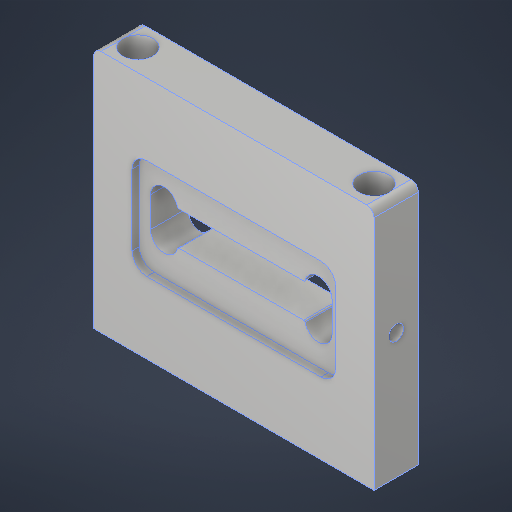
# Autodesk Inventor part: Spulenhalter Hinten Einzel
Saved by Autodesk Inventor 2025.2 (Build 292293000, 293)
## iProperties
Part Number: Spulenhalter Hinten Einzel
Material: Aluminium 6061
Document SubType Name: Modeling
Designer: rYan
Density: 2.7 g/cm^3
Appearance: Aluminium - flach
Mass: 16.9891 g
Surface Area: 44.1608 cm^2
Volume: 6.29226 cm^3
Author: rYan
Autodesk Inventor part; units mm, degrees
ref_plane "YZ Plane" through (0, 0, 0) normal (1, 0, 0) x (0, 1, 0)
ref_plane "XZ Plane" through (0, 0, 0) normal (0, 1, 0) x (-1, 0, 0)
ref_plane "XY Plane" through (0, 0, 0) normal (0, 0, 1) x (1, 0, 0)
sketch "Skizze1" plane through (0, 0, 0) normal (0, 1, 0) x (-1, 0, 0)
  line L0 (-19, 0) -> (-19, 30)
  line L1 (19, 30) -> (19, 0)
  line L2 (8.85, 11.45) -> (-8.85, 11.45)
  line L3 (-12.05, 11.45) -> (-12.05, 15.55)
  line L4 (-8.85, 15.55) -> (8.85, 15.55)
  line L5 (12.05, 15.55) -> (12.05, 11.45)
  arc A0 (12.05, 15.55) -> (8.85, 15.55) centre (10.45, 15.55) ccw
  arc A1 (8.85, 11.45) -> (12.05, 11.45) centre (10.45, 11.45) ccw
  arc A2 (-8.85, 15.55) -> (-12.05, 15.55) centre (-10.45, 15.55) ccw
  arc A3 (-12.05, 11.45) -> (-8.85, 11.45) centre (-10.45, 11.45) ccw
  line L6 (19, -3) -> (-19, -3)
  line L7 (-19, -3) -> (-19, 0)
  line L8 (19, 0) -> (19, -3)
  line L9 (0, 30) -> (19, 30)
  line L10 (19, 30) -> (-19, 30)
  arc A4 (-12.3, 11.45) -> (-8.617, 11.2) centre (-10.45, 11.45) ccw
  line L11 (-8.617, 11.2) -> (8.617, 11.2)
  arc A5 (8.617, 11.2) -> (12.3, 11.45) centre (10.45, 11.45) ccw
  line L12 (12.3, 11.45) -> (12.3, 15.55)
  arc A6 (12.3, 15.55) -> (8.617, 15.8) centre (10.45, 15.55) ccw
  line L13 (8.617, 15.8) -> (-8.617, 15.8)
  arc A7 (-8.617, 15.8) -> (-12.3, 15.55) centre (-10.45, 15.55) ccw
  line L14 (-12.3, 15.55) -> (-12.3, 11.45)
  line L15 (0, -3) -> (0, 30) construction
  point P0 (0, 13.5)
  point P1 (19, 0)
  point P2 (0, 13.5)
  dimension "d94" = 0.25
  constraints: 32 end point, 16 point on circle, 8 centre point, 6 parallel, 4 perpendicular, 4 tangent, 3 point on line, 2 horizontal, 2 midpoint, 6 other
  measures "d94" distance between parallel lines of L4 L13
extrude "Grundkörper" add sketch "Skizze1" along normal mid plane 6 contours L0 L10 L9 L1 L8 L6 L7
sketch "Skizze10" plane through (19, 3, -3) normal (0, 0, -1) x (-1, 0, 0)
  line L0 (-3.4, -3) -> (41.4, -3)
  line L1 (19, 19.4) -> (19, -25.4)
  point P0 (19, -3)
  point P1 (19, -3)
  point P2 (3, -3)
  point P3 (35, -3)
  dimension "d96" = 32
  constraints: 4 end point, 2 point on line, 1 symmetric about line
  measures "d96" distance of point (35, -3) point (3, -3)
hole "Fixierung" at (16, 0, -3) at (-16, 0, -3) direction (0, 0, 1) diameter 4.2 depth 8 tip angle 118
fillet "Rundung1" radius 1 2 edges at (-19, 0, 30) (19, 0, 30)
fillet "Rundung2" radius 0.2 4 edges at (-8.617, 0, 15.8) (8.617, 0, 15.8) (8.617, 0, 11.2) (-8.617, 0, 11.2)
sketch "Skizze13" plane through (0, -3, 0) normal (0, -1, 0) x (1, 0, 0)
  line L0 (-8.6611, 15.55) -> (8.6611, 15.55) construction
  line L1 (0, 15.55) -> (0, 11.45) construction
  line L2 (-8.6611, 11.45) -> (8.6611, 11.45) construction
  line L3 (-11.8, 6.7) -> (11.8, 6.7)
  line L4 (13.8, 8.7) -> (13.8, 18.3)
  line L5 (11.8, 20.3) -> (-11.8, 20.3)
  line L6 (-13.8, 18.3) -> (-13.8, 8.7)
  line L7 (-13.8, 6.7) -> (13.8, 20.3) construction
  line L8 (13.8, 6.7) -> (-13.8, 20.3) construction
  arc A0 (-11.8, 20.3) -> (-13.8, 18.3) centre (-11.8, 18.3) ccw
  arc A1 (-13.8, 8.7) -> (-11.8, 6.7) centre (-11.8, 8.7) ccw
  arc A2 (11.8, 6.7) -> (13.8, 8.7) centre (11.8, 8.7) ccw
  arc A3 (13.8, 18.3) -> (11.8, 20.3) centre (11.8, 18.3) ccw
  point P0 (0, 0)
  point P1 (0, 13.5)
  dimension "d125" = 27.6
  dimension "d126" = 13.6
  dimension "d127" = 2
  constraints: 14 end point, 8 point on circle, 8 point on line, 8 tangent, 5 midpoint, 4 centre point, 3 equal radius, 2 parallel, 1 horizontal, 1 perpendicular
  measures "d125" distance of L8.end L7.end
  measures "d126" distance of L7.end L8.start
  measures "d127" radius of A0
extrude "Tasche" cut sketch "Skizze13" against normal blind 1
sketch "Skizze11" plane through (19, -3, -3) normal (1, 0, 0) x (0, 0, -1)
  point P0 (-7, 3)
  point P1 (-17, 3)
hole "Federn" at (19, 0, 14) direction (-1, 0, 0) diameter 2 depth 4 tip angle 118
mirror "Spiegeln1" about plane through (0, 0, 0) normal (1, 0, 0) of "Federn"
sketch "Skizze12" plane through (-18, 3, 30) normal (0, 0, 1) x (1, 0, 0)
  line L0 (18, -3) -> (2, -3)
  line L1 (18, -3) -> (18, 0)
  line L2 (26.6611, 0) -> (9.3389, 0) projected
  point P0 (34, -3)
  dimension "d117" = 16
  constraints: 4 end point, 1 coincident, 1 horizontal, 1 midpoint, 1 symmetric about line
  measures "d117" distance of L0.start L0.end
hole "Platinenhalterung" at (-16, 0, 30) at (16, 0, 30) direction (0, 0, -1) diameter 4.1 depth 8 tip angle 118
